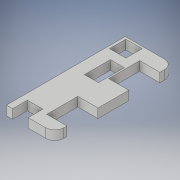
# Autodesk Inventor part: Charger_support
Saved by Autodesk Inventor 2017 (Build 210142000, 142)
## iProperties
Created: 2018-06-25
Part Number: Charger_support
Material: Generic
Document SubType Name: Modeling
Designer: Arthur
Density: 1 g/cm^3
Appearance: Default
Author: Arthur
Autodesk Inventor part; units mm, degrees
ref_plane "YZ Plane" through (0, 0, 0) normal (1, 0, 0) x (0, 1, 0)
ref_plane "XZ Plane" through (0, 0, 0) normal (0, 1, 0) x (-1, 0, 0)
ref_plane "XY Plane" through (0, 0, 0) normal (0, 0, 1) x (1, 0, 0)
sketch "Sketch1" plane through (0, 0, 0) normal (0, 1, 0) x (-1, 0, 0)
  line L0 (-14, 34.5) -> (12.387, 34.5)
  line L1 (12.387, 34.5) -> (12.387, -30.5)
  line L2 (12.387, -30.5) -> (-14, -30.5)
  line L3 (-14, -30.5) -> (-14, 34.5)
  dimension "d0" = 26.387
  dimension "d1" = 65
  constraints: 8 end point, 1 parallel
  measures "d0" distance of L1.end L2.end
  measures "d1" distance of L0.end L1.end
extrude "Extrusion1" add sketch "Sketch1" along normal blind 5
fillet "Fillet1" radius 5 2 edges at (14, 2.5, 34.5) (14, 2.5, -30.5)
sketch "Sketch2" plane through (0, 5, 0) normal (0, 1, 0) x (1, 0, 0)
  line L0 (-9, -34.5716) -> (-9, -26.4716)
  line L1 (-9, -26.4716) -> (-0.5, -26.4716)
  line L2 (-0.5, -26.4716) -> (-0.5, -34.5716)
  line L3 (-0.5, -34.5716) -> (-9, -34.5716)
  point P0 (0, 0)
  point P1 (-12.387, -34.5)
  dimension "d6" = 8.1
  dimension "d7" = 8.5
  constraints: 8 end point, 2 perpendicular
  measures "d6" distance of L0.start L0.end
  measures "d7" distance of L0.end L1.end
extrude "Extrusion2" cut sketch "Sketch2" against normal through all
sketch "Sketch3" plane through (0, 5, 0) normal (0, 1, 0) x (1, 0, 0)
  line L0 (14, -27.8288) -> (3, -27.8288)
  line L1 (3, -27.8288) -> (3, -10.8288)
  line L2 (3, -10.8288) -> (14, -10.8288)
  line L3 (14, -10.8288) -> (14, -27.8288)
  line L4 (14, 6.0005) -> (3, 6.0005)
  line L5 (3, 6.0005) -> (3, 23.0005)
  line L6 (3, 23.0005) -> (14, 23.0005)
  line L7 (14, 23.0005) -> (14, 6.0005)
  point P0 (0, 0)
  dimension "d12" = 11
  dimension "d13" = 17
  dimension "d22" = 11
  dimension "d23" = 17
  constraints: 16 end point, 4 parallel, 2 horizontal, 2 perpendicular
  measures "d12" distance of L1.end L2.end
  measures "d13" distance of L0.end L1.end
  measures "d22" distance of L5.end L7.start
  measures "d23" distance of L4.end L5.end
extrude "Extrusion3" cut sketch "Sketch3" against normal through all
sketch "Sketch4" plane through (0, 5, 0) normal (0, 1, 0) x (1, 0, 0)
  line L0 (14, 6.0005) -> (3, 6.0005) projected
  line L1 (3, 23.0005) -> (3, 6.0005) projected
  line L2 (2.1408, 15.4204) -> (-5.4822, 15.4204)
  line L3 (-5.4822, 15.4204) -> (-5.4822, 1.2634)
  line L4 (-5.4822, 1.2634) -> (2.1408, 1.2634)
  line L5 (2.1408, 1.2634) -> (2.1408, 15.4204)
  line L6 (-12.387, 30.5) -> (-12.387, -34.5) projected
  line L7 (-10.912, 29.3102) -> (-2, 29.3102)
  line L8 (-2, 29.3102) -> (-2, 20.3982)
  line L9 (-2, 20.3982) -> (-10.912, 20.3982)
  line L10 (-10.912, 20.3982) -> (-10.912, 29.3102)
  point P0 (0, 0)
  dimension "d29" = 7.623
  dimension "d30" = 14.157
  dimension "d33" = 8.912
  dimension "d34" = 8.912
  constraints: 16 end point, 4 parallel, 2 horizontal, 2 perpendicular
  measures "d29" distance of L4.end L3.end
  measures "d30" distance of L3.end L2.end
  measures "d33" distance of L8.end L9.end
  measures "d34" distance of L7.end L8.end
extrude "Extrusion4" cut sketch "Sketch4" against normal through all
body "Solid1"
